Autodesk Inventor part; units mm, degrees
(part 2 of 3)
sketch "Sketch72" plane through (-75.2, 2, 54) normal (0, 1, 0) x (1, 0, 0)
  line L0 (165.4, 13.35) -> (165.4, 23.35) projected
  line L1 (17.3, 78.3) -> (17.3, 97) projected
  line L2 (17.3, 97) -> (-15, 97) projected
  line L3 (-15, 97) -> (-15, 78.3) projected
  line L4 (-15, 78.3) -> (17.3, 78.3) projected
  line L5 (12.24, 7) -> (12.24, 22.5) projected
  line L6 (12.24, 22.5) -> (-7, 22.5) projected
  line L7 (-7, 22.5) -> (-7, 7) projected
  line L8 (-7, 7) -> (12.24, 7) projected
  line L9 (150.4, 110.9) -> (150.4, 105.9) projected
  line L10 (150.4, 105.9) -> (130.4, 105.9) projected
  line L11 (130.4, 105.9) -> (130.4, 110.9) projected
  line L12 (130.4, 110.9) -> (150.4, 110.9) projected
  circle A0 centre (124.902, 56.094) radius 1 projected
  circle A1 centre (89.469, 56.094) radius 1 projected
  circle A2 centre (89.469, 91.502) radius 1 projected
  circle A3 centre (124.902, 91.502) radius 1 projected
  circle A4 centre (104.2, 13.0337) radius 1.5 projected
  circle A5 centre (46.2, 13.0337) radius 1.5 projected
  circle A6 centre (46.2, 36.0337) radius 1.5 projected
  circle A7 centre (104.2, 36.0337) radius 1.5 projected
  circle A8 centre (104.2, 13.0337) radius 3 projected
  circle A9 centre (46.2, 13.0337) radius 3 projected
  circle A10 centre (104.2, 36.0337) radius 3 projected
  circle A11 centre (46.2, 36.0337) radius 3 projected
  circle A12 centre (-2.46, 5.26) radius 1.275 projected
  circle A13 centre (7.7, 5.26) radius 1.275 projected
  line L13 (91.971, 89) -> (91.971, 58.596) projected
  line L14 (91.971, 58.596) -> (102, 58.596) projected
  line L15 (102, 58.596) -> (102, 39.596) projected
  line L16 (102, 39.596) -> (110.4, 39.596) projected
  line L17 (110.4, 39.596) -> (110.4, -1.404) projected
  line L18 (110.4, -1.404) -> (122.4, -1.404) projected
  line L19 (122.4, -1.404) -> (122.4, 56.094) projected
  circle A14 centre (124.902, 56.094) radius 2.502 projected
  line L20 (122.4, 56.094) -> (122.4, 89) projected
  line L21 (122.4, 89) -> (91.971, 89) projected
  circle A15 centre (89.469, 56.094) radius 2.502 projected
  circle A16 centre (124.902, 91.502) radius 2.502 projected
  circle A17 centre (89.469, 91.502) radius 2.502 projected
  line L22 (157.4, 72.95) -> (162.4, 72.95) projected
  line L23 (162.4, 72.95) -> (162.4, 32.95) projected
  line L24 (157.4, 32.95) -> (157.4, 72.95) projected
  line L25 (-7, 72.95) -> (-7, 32.95) projected
  line L26 (-12, 32.95) -> (-12, 72.95) projected
  line L27 (-12, 72.95) -> (-7, 72.95) projected
  line L28 (20, 110.9) -> (20, 105.9) projected
  line L29 (20, 105.9) -> (0, 105.9) projected
  line L30 (0, 105.9) -> (0, 110.9) projected
  line L31 (0, 110.9) -> (20, 110.9) projected
  line L32 (137.4, 37) -> (137.4, 34) projected
  line L33 (137.4, 34) -> (134.2775, 34) projected
  line L34 (134.2775, 34) -> (134.2775, 37) projected
  line L35 (134.2775, 37) -> (137.4, 37) projected
  line L36 (137.4, 37) -> (140.5225, 37) projected
  line L37 (140.5225, 37) -> (140.5225, 34) projected
  line L38 (140.5225, 34) -> (137.4, 34) projected
  arc A18 (-12, 116) -> (-17, 111) centre (-12, 111) ccw projected
  line L39 (-12, 116) -> (36.4, 116) projected
  line L40 (36.4, 116) -> (36.4, 115.5) projected
  line L41 (36.4, 115.5) -> (37, 115.5) projected
  line L42 (37, 115.5) -> (50.2, 115.5) projected
  line L43 (50.2, 115.5) -> (50.8, 115.5) projected
  line L44 (50.8, 115.5) -> (50.8, 116) projected
  line L45 (50.8, 116) -> (60.4, 116) projected
  line L46 (60.4, 116) -> (60.4, 115.5) projected
  line L47 (60.4, 115.5) -> (61, 115.5) projected
  line L48 (61, 115.5) -> (74.2, 115.5) projected
  line L49 (74.2, 115.5) -> (74.8, 115.5) projected
  line L50 (74.8, 115.5) -> (74.8, 116) projected
  line L51 (74.8, 116) -> (162.4, 116) projected
  arc A19 (167.4, 111) -> (162.4, 116) centre (162.4, 111) ccw projected
  line L52 (167.4, 111) -> (167.4, -3) projected
  arc A20 (162.4, -8) -> (167.4, -3) centre (162.4, -3) ccw projected
  line L53 (162.4, -8) -> (-12, -8) projected
  arc A21 (-17, -3) -> (-12, -8) centre (-12, -3) ccw projected
  line L54 (-17, -3) -> (-17, 111) projected
  line L55 (37, 115.5) -> (37, 102.8) projected
  line L56 (37, 102.8) -> (35.5, 102.8) projected
  line L57 (35.5, 102.8) -> (35.5, 112) projected
  line L58 (35.5, 112) -> (34, 112) projected
  line L59 (34, 112) -> (34, 114) projected
  line L60 (34, 114) -> (22, 114) projected
  line L61 (22, 114) -> (22, 112) projected
  line L62 (22, 112) -> (-12, 112) projected
  arc A22 (-12, 112) -> (-13, 111) centre (-12, 111) ccw projected
  line L63 (-13, 111) -> (-13, 100) projected
  line L64 (-13, 100) -> (19.3, 100) projected
  line L65 (19.3, 100) -> (19.3, 75.3) projected
  line L66 (19.3, 75.3) -> (-13, 75.3) projected
  line L67 (-13, 75.3) -> (-13, 77.3) projected
  line L68 (50.2, 102.8) -> (50.2, 115.5) projected
  line L69 (51.7, 102.8) -> (50.2, 102.8) projected
  line L70 (51.7, 112) -> (51.7, 102.8) projected
  line L71 (59.5, 112) -> (51.7, 112) projected
  line L72 (59.5, 102.8) -> (59.5, 112) projected
  line L73 (61, 102.8) -> (59.5, 102.8) projected
  line L74 (61, 115.5) -> (61, 102.8) projected
  line L75 (74.2, 102.8) -> (74.2, 115.5) projected
  line L76 (75.7, 102.8) -> (74.2, 102.8) projected
  line L77 (75.7, 112) -> (75.7, 102.8) projected
  line L78 (116.4, 112) -> (75.7, 112) projected
  line L79 (116.4, 114) -> (116.4, 112) projected
  line L80 (128.4, 114) -> (116.4, 114) projected
  line L81 (128.4, 112) -> (128.4, 114) projected
  line L82 (162.4, 112) -> (128.4, 112) projected
  arc A23 (163.4, 111) -> (162.4, 112) centre (162.4, 111) ccw projected
  line L83 (163.4, -3) -> (163.4, 111) projected
  arc A24 (162.4, -4) -> (163.4, -3) centre (162.4, -3) ccw projected
  line L84 (150.4, -4) -> (162.4, -4) projected
  line L85 (150.4, 0) -> (150.4, -4) projected
  line L86 (130.4, 0) -> (150.4, 0) projected
  line L87 (130.4, -4) -> (130.4, 0) projected
  line L88 (128.4, -4) -> (130.4, -4) projected
  line L89 (128.4, -6) -> (128.4, -4) projected
  line L90 (116.4, -6) -> (128.4, -6) projected
  line L91 (116.4, -4) -> (116.4, -6) projected
  line L92 (34, -4) -> (116.4, -4) projected
  line L93 (34, -4) -> (22, -4) projected
  line L94 (20, -4) -> (22, -4) projected
  line L95 (20, 0) -> (20, -4) projected
  line L96 (0, 0) -> (20, 0) projected
  line L97 (0, -4) -> (0, 0) projected
  line L98 (-12, -4) -> (0, -4) projected
  arc A25 (-13, -3) -> (-12, -4) centre (-12, -3) ccw projected
  line L99 (-13, 48) -> (-13, -3) projected
  line L100 (-13, 48) -> (-13, 60) projected
  line L101 (-13, 75.3) -> (-13, 60) projected
  line L102 (22, 112) -> (34, 112) projected
  line L103 (-13, 98) -> (-13, 100) projected
  line L104 (116.4, 112) -> (128.4, 112) projected
  line L105 (128.4, -4) -> (116.4, -4) projected
  line L106 (34, -6) -> (34, -4) projected
  line L107 (22, -6) -> (34, -6) projected
  line L108 (22, -4) -> (22, -6) projected
  line L109 (-15, 48) -> (-13, 48) projected
  line L110 (-15, 60) -> (-15, 48) projected
  line L111 (-13, 60) -> (-15, 60) projected
  line L112 (163.4, 111) -> (163.4, -3) projected
  line L113 (167.4, 13.35) -> (165.4, 13.35) projected
  line L114 (163.4, 13.35) -> (163.4, 30.0547)
  line L115 (17.3, 78.3) -> (17.3, 97) projected
  line L116 (17.3, 97) -> (-15, 97) projected
  line L117 (-15, 97) -> (-15, 78.3) projected
  line L118 (-15, 78.3) -> (17.3, 78.3) projected
  line L119 (150.4, 110.9) -> (150.4, 105.9) projected
  line L120 (150.4, 105.9) -> (130.4, 105.9) projected
  line L121 (130.4, 105.9) -> (130.4, 110.9) projected
  line L122 (130.4, 110.9) -> (150.4, 110.9) projected
  circle A26 centre (124.902, 56.094) radius 1 projected
  circle A27 centre (89.469, 56.094) radius 1 projected
  circle A28 centre (89.469, 91.502) radius 1 projected
  circle A29 centre (124.902, 91.502) radius 1 projected
  circle A30 centre (104.2, 13.0337) radius 1.5 projected
  circle A31 centre (46.2, 13.0337) radius 1.5 projected
  circle A32 centre (46.2, 36.0337) radius 1.5 projected
  circle A33 centre (104.2, 36.0337) radius 1.5 projected
  circle A34 centre (104.2, 13.0337) radius 3 projected
  circle A35 centre (46.2, 13.0337) radius 3 projected
  circle A36 centre (104.2, 36.0337) radius 3 projected
  circle A37 centre (46.2, 36.0337) radius 3 projected
  circle A38 centre (-2.46, 5.26) radius 1.275 projected
  circle A39 centre (7.7, 5.26) radius 1.275 projected
  line L123 (91.971, 89) -> (91.971, 58.596) projected
  line L124 (91.971, 58.596) -> (102, 58.596) projected
  line L125 (102, 58.596) -> (102, 39.596) projected
  line L126 (102, 39.596) -> (110.4, 39.596) projected
  line L127 (110.4, 39.596) -> (110.4, -1.404) projected
  line L128 (110.4, -1.404) -> (122.4, -1.404) projected
  line L129 (122.4, -1.404) -> (122.4, 56.094) projected
  circle A40 centre (124.902, 56.094) radius 2.502 projected
  line L130 (122.4, 56.094) -> (122.4, 89) projected
  line L131 (122.4, 89) -> (91.971, 89) projected
  circle A41 centre (89.469, 56.094) radius 2.502 projected
  circle A42 centre (124.902, 91.502) radius 2.502 projected
  circle A43 centre (89.469, 91.502) radius 2.502 projected
  line L132 (157.4, 72.95) -> (162.4, 72.95) projected
  line L133 (162.4, 72.95) -> (162.4, 32.95) projected
  line L134 (-12, 32.95) -> (-12, 72.95) projected
  line L135 (-12, 72.95) -> (-7, 72.95) projected
  line L136 (20, 110.9) -> (20, 105.9) projected
  line L137 (20, 105.9) -> (0, 105.9) projected
  line L138 (0, 105.9) -> (0, 110.9) projected
  line L139 (0, 110.9) -> (20, 110.9) projected
  arc A44 (-12, 116) -> (-17, 111) centre (-12, 111) ccw projected
  line L140 (-12, 116) -> (36.4, 116) projected
  line L141 (36.4, 116) -> (36.4, 115.5) projected
  line L142 (36.4, 115.5) -> (37, 115.5) projected
  line L143 (37, 115.5) -> (50.2, 115.5) projected
  line L144 (50.8, 116) -> (60.4, 116) projected
  line L145 (60.4, 116) -> (60.4, 115.5) projected
  line L146 (60.4, 115.5) -> (61, 115.5) projected
  line L147 (61, 115.5) -> (74.2, 115.5) projected
  line L148 (74.8, 116) -> (162.4, 116) projected
  arc A45 (167.4, 111) -> (162.4, 116) centre (162.4, 111) ccw projected
  line L149 (167.4, 111) -> (167.4, -3) projected
  arc A46 (162.4, -8) -> (167.4, -3) centre (162.4, -3) ccw projected
  line L150 (162.4, -8) -> (-12, -8) projected
  arc A47 (-17, -3) -> (-12, -8) centre (-12, -3) ccw projected
  line L151 (-17, -3) -> (-17, 111) projected
  line L152 (37, 115.5) -> (37, 102.8) projected
  line L153 (37, 102.8) -> (35.5, 102.8) projected
  line L154 (35.5, 102.8) -> (35.5, 112) projected
  line L155 (35.5, 112) -> (34, 112) projected
  line L156 (34, 112) -> (34, 114) projected
  line L157 (34, 114) -> (22, 114) projected
  line L158 (22, 114) -> (22, 112) projected
  line L159 (22, 112) -> (-12, 112) projected
  arc A48 (-12, 112) -> (-13, 111) centre (-12, 111) ccw projected
  line L160 (-13, 111) -> (-13, 100) projected
  line L161 (-13, 100) -> (19.3, 100) projected
  line L162 (19.3, 100) -> (19.3, 75.3) projected
  line L163 (19.3, 75.3) -> (-13, 75.3) projected
  line L164 (-13, 75.3) -> (-13, 77.3) projected
  line L165 (59.5, 112) -> (51.7, 112) projected
  line L166 (59.5, 102.8) -> (59.5, 112) projected
  line L167 (61, 102.8) -> (59.5, 102.8) projected
  line L168 (61, 115.5) -> (61, 102.8) projected
  line L169 (116.4, 112) -> (75.7, 112) projected
  line L170 (116.4, 114) -> (116.4, 112) projected
  line L171 (128.4, 114) -> (116.4, 114) projected
  line L172 (128.4, 112) -> (128.4, 114) projected
  line L173 (162.4, 112) -> (128.4, 112) projected
  arc A49 (163.4, 111) -> (162.4, 112) centre (162.4, 111) ccw projected
  line L174 (163.4, -3) -> (163.4, 111) projected
  arc A50 (162.4, -4) -> (163.4, -3) centre (162.4, -3) ccw projected
  line L175 (150.4, -4) -> (162.4, -4) projected
  line L176 (150.4, 0) -> (150.4, -4) projected
  line L177 (130.4, 0) -> (150.4, 0) projected
  line L178 (130.4, -4) -> (130.4, 0) projected
  line L179 (128.4, -4) -> (130.4, -4) projected
  line L180 (128.4, -6) -> (128.4, -4) projected
  line L181 (116.4, -6) -> (128.4, -6) projected
  line L182 (116.4, -4) -> (116.4, -6) projected
  line L183 (34, -4) -> (116.4, -4) projected
  line L184 (34, -4) -> (22, -4) projected
  line L185 (20, -4) -> (22, -4) projected
  line L186 (20, 0) -> (20, -4) projected
  line L187 (0, 0) -> (20, 0) projected
  line L188 (0, -4) -> (0, 0) projected
  line L189 (-12, -4) -> (0, -4) projected
  arc A51 (-13, -3) -> (-12, -4) centre (-12, -3) ccw projected
  line L190 (-13, 48) -> (-13, -3) projected
  line L191 (-13, 48) -> (-13, 60) projected
  line L192 (-13, 75.3) -> (-13, 60) projected
  line L193 (22, 112) -> (34, 112) projected
  line L194 (-13, 98) -> (-13, 100) projected
  line L195 (116.4, 112) -> (128.4, 112) projected
  line L196 (128.4, -4) -> (116.4, -4) projected
  line L197 (34, -6) -> (34, -4) projected
  line L198 (22, -6) -> (34, -6) projected
  line L199 (22, -4) -> (22, -6) projected
  line L200 (-15, 48) -> (-13, 48) projected
  line L201 (-15, 60) -> (-15, 48) projected
  line L202 (-13, 60) -> (-15, 60) projected
  line L203 (17.3, 78.3) -> (17.3, 97) projected
  line L204 (17.3, 97) -> (-15, 97) projected
  line L205 (-15, 97) -> (-15, 78.3) projected
  line L206 (-15, 78.3) -> (17.3, 78.3) projected
  line L207 (150.4, 110.9) -> (150.4, 105.9) projected
  line L208 (150.4, 105.9) -> (130.4, 105.9) projected
  line L209 (130.4, 105.9) -> (130.4, 110.9) projected
  line L210 (130.4, 110.9) -> (150.4, 110.9) projected
  circle A52 centre (124.902, 56.094) radius 1 projected
  circle A53 centre (89.469, 56.094) radius 1 projected
  circle A54 centre (89.469, 91.502) radius 1 projected
  circle A55 centre (124.902, 91.502) radius 1 projected
  circle A56 centre (104.2, 13.0337) radius 1.5 projected
  circle A57 centre (46.2, 13.0337) radius 1.5 projected
  circle A58 centre (46.2, 36.0337) radius 1.5 projected
  circle A59 centre (104.2, 36.0337) radius 1.5 projected
  circle A60 centre (104.2, 13.0337) radius 3 projected
  circle A61 centre (46.2, 13.0337) radius 3 projected
  circle A62 centre (104.2, 36.0337) radius 3 projected
  circle A63 centre (46.2, 36.0337) radius 3 projected
  circle A64 centre (-2.46, 5.26) radius 1.275 projected
  circle A65 centre (7.7, 5.26) radius 1.275 projected
  line L211 (91.971, 89) -> (91.971, 58.596) projected
  line L212 (91.971, 58.596) -> (102, 58.596) projected
  line L213 (102, 58.596) -> (102, 39.596) projected
  line L214 (102, 39.596) -> (110.4, 39.596) projected
  line L215 (110.4, 39.596) -> (110.4, -1.404) projected
  line L216 (110.4, -1.404) -> (122.4, -1.404) projected
  line L217 (122.4, -1.404) -> (122.4, 56.094) projected
  circle A66 centre (124.902, 56.094) radius 2.502 projected
  line L218 (122.4, 56.094) -> (122.4, 89) projected
  line L219 (122.4, 89) -> (91.971, 89) projected
  circle A67 centre (89.469, 56.094) radius 2.502 projected
  circle A68 centre (124.902, 91.502) radius 2.502 projected
  circle A69 centre (89.469, 91.502) radius 2.502 projected
  line L220 (157.4, 72.95) -> (162.4, 72.95) projected
  line L221 (162.4, 72.95) -> (162.4, 32.95) projected
  line L222 (-12, 32.95) -> (-12, 72.95) projected
  line L223 (-12, 72.95) -> (-7, 72.95) projected
  line L224 (20, 110.9) -> (20, 105.9) projected
  line L225 (20, 105.9) -> (0, 105.9) projected
  line L226 (0, 105.9) -> (0, 110.9) projected
  line L227 (0, 110.9) -> (20, 110.9) projected
  arc A70 (-12, 116) -> (-17, 111) centre (-12, 111) ccw projected
  line L228 (-12, 116) -> (36.4, 116) projected
  line L229 (36.4, 116) -> (36.4, 115.5) projected
  line L230 (36.4, 115.5) -> (37, 115.5) projected
  line L231 (37, 115.5) -> (50.2, 115.5) projected
  line L232 (50.8, 116) -> (60.4, 116) projected
  line L233 (60.4, 116) -> (60.4, 115.5) projected
  line L234 (60.4, 115.5) -> (61, 115.5) projected
  line L235 (61, 115.5) -> (74.2, 115.5) projected
  line L236 (74.8, 116) -> (162.4, 116) projected
  arc A71 (167.4, 111) -> (162.4, 116) centre (162.4, 111) ccw projected
  line L237 (167.4, 111) -> (167.4, -3) projected
  arc A72 (162.4, -8) -> (167.4, -3) centre (162.4, -3) ccw projected
  line L238 (162.4, -8) -> (-12, -8) projected
  arc A73 (-17, -3) -> (-12, -8) centre (-12, -3) ccw projected
  line L239 (-17, -3) -> (-17, 111) projected
  line L240 (37, 115.5) -> (37, 102.8) projected
  line L241 (37, 102.8) -> (35.5, 102.8) projected
  line L242 (35.5, 102.8) -> (35.5, 112) projected
  line L243 (35.5, 112) -> (34, 112) projected
  line L244 (34, 112) -> (34, 114) projected
  line L245 (34, 114) -> (22, 114) projected
  line L246 (22, 114) -> (22, 112) projected
  line L247 (22, 112) -> (-12, 112) projected
  arc A74 (-12, 112) -> (-13, 111) centre (-12, 111) ccw projected
  line L248 (-13, 111) -> (-13, 100) projected
  line L249 (-13, 100) -> (19.3, 100) projected
  line L250 (19.3, 100) -> (19.3, 75.3) projected
  line L251 (19.3, 75.3) -> (-13, 75.3) projected
  line L252 (-13, 75.3) -> (-13, 77.3) projected
  line L253 (59.5, 112) -> (51.7, 112) projected
  line L254 (59.5, 102.8) -> (59.5, 112) projected
  line L255 (61, 102.8) -> (59.5, 102.8) projected
  line L256 (61, 115.5) -> (61, 102.8) projected
  line L257 (116.4, 112) -> (75.7, 112) projected
  line L258 (116.4, 114) -> (116.4, 112) projected
  line L259 (128.4, 114) -> (116.4, 114) projected
  line L260 (128.4, 112) -> (128.4, 114) projected
  line L261 (162.4, 112) -> (128.4, 112) projected
  arc A75 (163.4, 111) -> (162.4, 112) centre (162.4, 111) ccw projected
  line L262 (163.4, -3) -> (163.4, 111) projected
  arc A76 (162.4, -4) -> (163.4, -3) centre (162.4, -3) ccw projected
  line L263 (150.4, -4) -> (162.4, -4) projected
  line L264 (150.4, 0) -> (150.4, -4) projected
  line L265 (130.4, 0) -> (150.4, 0) projected
  line L266 (130.4, -4) -> (130.4, 0) projected
  line L267 (128.4, -4) -> (130.4, -4) projected
  line L268 (128.4, -6) -> (128.4, -4) projected
  line L269 (116.4, -6) -> (128.4, -6) projected
  line L270 (116.4, -4) -> (116.4, -6) projected
  line L271 (34, -4) -> (116.4, -4) projected
  line L272 (34, -4) -> (22, -4) projected
  line L273 (20, -4) -> (22, -4) projected
  line L274 (20, 0) -> (20, -4) projected
  line L275 (0, 0) -> (20, 0) projected
  line L276 (0, -4) -> (0, 0) projected
  line L277 (-12, -4) -> (0, -4) projected
  arc A77 (-13, -3) -> (-12, -4) centre (-12, -3) ccw projected
  line L278 (-13, 48) -> (-13, -3) projected
  line L279 (-13, 48) -> (-13, 60) projected
  line L280 (-13, 75.3) -> (-13, 60) projected
  line L281 (22, 112) -> (34, 112) projected
  line L282 (-13, 98) -> (-13, 100) projected
  line L283 (116.4, 112) -> (128.4, 112) projected
  line L284 (128.4, -4) -> (116.4, -4) projected
  line L285 (34, -6) -> (34, -4) projected
  line L286 (22, -6) -> (34, -6) projected
  line L287 (22, -4) -> (22, -6) projected
  line L288 (-15, 48) -> (-13, 48) projected
  line L289 (-15, 60) -> (-15, 48) projected
  line L290 (-13, 60) -> (-15, 60) projected
  line L291 (17.3, 78.3) -> (17.3, 97) projected
  line L292 (17.3, 97) -> (-15, 97) projected
  line L293 (-15, 97) -> (-15, 78.3) projected
  line L294 (-15, 78.3) -> (17.3, 78.3) projected
  line L295 (150.4, 110.9) -> (150.4, 105.9) projected
  line L296 (150.4, 105.9) -> (130.4, 105.9) projected
  line L297 (130.4, 105.9) -> (130.4, 110.9) projected
  line L298 (130.4, 110.9) -> (150.4, 110.9) projected
  circle A78 centre (124.902, 56.094) radius 1 projected
  circle A79 centre (89.469, 56.094) radius 1 projected
  circle A80 centre (89.469, 91.502) radius 1 projected
  circle A81 centre (124.902, 91.502) radius 1 projected
  circle A82 centre (104.2, 13.0337) radius 1.5 projected
  circle A83 centre (46.2, 13.0337) radius 1.5 projected
  circle A84 centre (46.2, 36.0337) radius 1.5 projected
  circle A85 centre (104.2, 36.0337) radius 1.5 projected
  circle A86 centre (104.2, 13.0337) radius 3 projected
  circle A87 centre (46.2, 13.0337) radius 3 projected
  circle A88 centre (104.2, 36.0337) radius 3 projected
  circle A89 centre (46.2, 36.0337) radius 3 projected
  circle A90 centre (-2.46, 5.26) radius 1.275 projected
  circle A91 centre (7.7, 5.26) radius 1.275 projected
  line L299 (91.971, 89) -> (91.971, 58.596) projected
  line L300 (91.971, 58.596) -> (102, 58.596) projected
  line L301 (102, 58.596) -> (102, 39.596) projected
  line L302 (102, 39.596) -> (110.4, 39.596) projected
  line L303 (110.4, 39.596) -> (110.4, -1.404) projected
  line L304 (110.4, -1.404) -> (122.4, -1.404) projected
  line L305 (122.4, -1.404) -> (122.4, 56.094) projected
  circle A92 centre (124.902, 56.094) radius 2.502 projected
  line L306 (122.4, 56.094) -> (122.4, 89) projected
  line L307 (122.4, 89) -> (91.971, 89) projected
  circle A93 centre (89.469, 56.094) radius 2.502 projected
  circle A94 centre (124.902, 91.502) radius 2.502 projected
  circle A95 centre (89.469, 91.502) radius 2.502 projected
  line L308 (157.4, 72.95) -> (162.4, 72.95) projected
  line L309 (162.4, 72.95) -> (162.4, 32.95) projected
  line L310 (-12, 32.95) -> (-12, 72.95) projected
  line L311 (-12, 72.95) -> (-7, 72.95) projected
  line L312 (20, 110.9) -> (20, 105.9) projected
  line L313 (20, 105.9) -> (0, 105.9) projected
  line L314 (0, 105.9) -> (0, 110.9) projected
  line L315 (0, 110.9) -> (20, 110.9) projected
  arc A96 (-12, 116) -> (-17, 111) centre (-12, 111) ccw projected
  line L316 (-12, 116) -> (36.4, 116) projected
  line L317 (36.4, 116) -> (36.4, 115.5) projected
  line L318 (36.4, 115.5) -> (37, 115.5) projected
  line L319 (37, 115.5) -> (50.2, 115.5) projected
  line L320 (50.8, 116) -> (60.4, 116) projected
  line L321 (60.4, 116) -> (60.4, 115.5) projected
  line L322 (60.4, 115.5) -> (61, 115.5) projected
  line L323 (61, 115.5) -> (74.2, 115.5) projected
  line L324 (74.8, 116) -> (162.4, 116) projected
  arc A97 (167.4, 111) -> (162.4, 116) centre (162.4, 111) ccw projected
  line L325 (167.4, 111) -> (167.4, -3) projected
  arc A98 (162.4, -8) -> (167.4, -3) centre (162.4, -3) ccw projected
  line L326 (162.4, -8) -> (-12, -8) projected
  arc A99 (-17, -3) -> (-12, -8) centre (-12, -3) ccw projected
  line L327 (-17, -3) -> (-17, 111) projected
  line L328 (37, 115.5) -> (37, 102.8) projected
  line L329 (37, 102.8) -> (35.5, 102.8) projected
  line L330 (35.5, 102.8) -> (35.5, 112) projected
  line L331 (35.5, 112) -> (34, 112) projected
  line L332 (34, 112) -> (34, 114) projected
  line L333 (34, 114) -> (22, 114) projected
  line L334 (22, 114) -> (22, 112) projected
  line L335 (22, 112) -> (-12, 112) projected
  arc A100 (-12, 112) -> (-13, 111) centre (-12, 111) ccw projected
  line L336 (-13, 111) -> (-13, 100) projected
  line L337 (-13, 100) -> (19.3, 100) projected
  line L338 (19.3, 100) -> (19.3, 75.3) projected
  line L339 (19.3, 75.3) -> (-13, 75.3) projected
  line L340 (-13, 75.3) -> (-13, 77.3) projected
  line L341 (59.5, 112) -> (51.7, 112) projected
  line L342 (59.5, 102.8) -> (59.5, 112) projected
  line L343 (61, 102.8) -> (59.5, 102.8) projected
  line L344 (61, 115.5) -> (61, 102.8) projected
  line L345 (116.4, 112) -> (75.7, 112) projected
  line L346 (116.4, 114) -> (116.4, 112) projected
  line L347 (128.4, 114) -> (116.4, 114) projected
  line L348 (128.4, 112) -> (128.4, 114) projected
  line L349 (162.4, 112) -> (128.4, 112) projected
  arc A101 (163.4, 111) -> (162.4, 112) centre (162.4, 111) ccw projected
  line L350 (163.4, -3) -> (163.4, 111) projected
  arc A102 (162.4, -4) -> (163.4, -3) centre (162.4, -3) ccw projected
  line L351 (150.4, -4) -> (162.4, -4) projected
  line L352 (150.4, 0) -> (150.4, -4) projected
  line L353 (130.4, 0) -> (150.4, 0) projected
  line L354 (130.4, -4) -> (130.4, 0) projected
  line L355 (128.4, -4) -> (130.4, -4) projected
  line L356 (128.4, -6) -> (128.4, -4) projected
  line L357 (116.4, -6) -> (128.4, -6) projected
  line L358 (116.4, -4) -> (116.4, -6) projected
  line L359 (34, -4) -> (116.4, -4) projected
  line L360 (34, -4) -> (22, -4) projected
  line L361 (20, -4) -> (22, -4) projected
  line L362 (20, 0) -> (20, -4) projected
  line L363 (0, 0) -> (20, 0) projected
  line L364 (0, -4) -> (0, 0) projected
  line L365 (-12, -4) -> (0, -4) projected
  arc A103 (-13, -3) -> (-12, -4) centre (-12, -3) ccw projected
  line L366 (-13, 48) -> (-13, -3) projected
  line L367 (-13, 48) -> (-13, 60) projected
  line L368 (-13, 75.3) -> (-13, 60) projected
  line L369 (22, 112) -> (34, 112) projected
  line L370 (-13, 98) -> (-13, 100) projected
  line L371 (116.4, 112) -> (128.4, 112) projected
  line L372 (128.4, -4) -> (116.4, -4) projected
  line L373 (34, -6) -> (34, -4) projected
  line L374 (22, -6) -> (34, -6) projected
  line L375 (22, -4) -> (22, -6) projected
  line L376 (-15, 48) -> (-13, 48) projected
  line L377 (-15, 60) -> (-15, 48) projected
  line L378 (-13, 60) -> (-15, 60) projected
  line L379 (17.3, 78.3) -> (17.3, 97) projected
  line L380 (17.3, 97) -> (-15, 97) projected
  line L381 (-15, 97) -> (-15, 78.3) projected
  line L382 (-15, 78.3) -> (17.3, 78.3) projected
  line L383 (150.4, 110.9) -> (150.4, 105.9) projected
  line L384 (150.4, 105.9) -> (130.4, 105.9) projected
  line L385 (130.4, 105.9) -> (130.4, 110.9) projected
  line L386 (130.4, 110.9) -> (150.4, 110.9) projected
  circle A104 centre (124.902, 56.094) radius 1 projected
  circle A105 centre (89.469, 56.094) radius 1 projected
  circle A106 centre (89.469, 91.502) radius 1 projected
  circle A107 centre (124.902, 91.502) radius 1 projected
  circle A108 centre (104.2, 13.0337) radius 1.5 projected
  circle A109 centre (46.2, 13.0337) radius 1.5 projected
  circle A110 centre (46.2, 36.0337) radius 1.5 projected
  circle A111 centre (104.2, 36.0337) radius 1.5 projected
  circle A112 centre (104.2, 13.0337) radius 3 projected
  circle A113 centre (46.2, 13.0337) radius 3 projected
  circle A114 centre (104.2, 36.0337) radius 3 projected
  circle A115 centre (46.2, 36.0337) radius 3 projected
  circle A116 centre (-2.46, 5.26) radius 1.275 projected
  circle A117 centre (7.7, 5.26) radius 1.275 projected
  line L387 (91.971, 89) -> (91.971, 58.596) projected
  line L388 (91.971, 58.596) -> (102, 58.596) projected
  line L389 (102, 58.596) -> (102, 39.596) projected
  line L390 (102, 39.596) -> (110.4, 39.596) projected
  line L391 (110.4, 39.596) -> (110.4, -1.404) projected
  line L392 (110.4, -1.404) -> (122.4, -1.404) projected
  line L393 (122.4, -1.404) -> (122.4, 56.094) projected
  circle A118 centre (124.902, 56.094) radius 2.502 projected
  line L394 (122.4, 56.094) -> (122.4, 89) projected
  line L395 (122.4, 89) -> (91.971, 89) projected
  circle A119 centre (89.469, 56.094) radius 2.502 projected
  circle A120 centre (124.902, 91.502) radius 2.502 projected
  circle A121 centre (89.469, 91.502) radius 2.502 projected
  line L396 (157.4, 72.95) -> (162.4, 72.95) projected
  line L397 (162.4, 72.95) -> (162.4, 32.95) projected
  line L398 (-12, 32.95) -> (-12, 72.95) projected
  line L399 (-12, 72.95) -> (-7, 72.95) projected
  line L400 (20, 110.9) -> (20, 105.9) projected
  line L401 (20, 105.9) -> (0, 105.9) projected
  line L402 (0, 105.9) -> (0, 110.9) projected
  line L403 (0, 110.9) -> (20, 110.9) projected
  arc A122 (-12, 116) -> (-17, 111) centre (-12, 111) ccw projected
  line L404 (-12, 116) -> (36.4, 116) projected
  line L405 (36.4, 116) -> (36.4, 115.5) projected
  line L406 (36.4, 115.5) -> (37, 115.5) projected
  line L407 (37, 115.5) -> (50.2, 115.5) projected
  line L408 (50.8, 116) -> (60.4, 116) projected
  line L409 (60.4, 116) -> (60.4, 115.5) projected
  line L410 (60.4, 115.5) -> (61, 115.5) projected
  line L411 (61, 115.5) -> (74.2, 115.5) projected
  line L412 (74.8, 116) -> (162.4, 116) projected
  arc A123 (167.4, 111) -> (162.4, 116) centre (162.4, 111) ccw projected
  line L413 (167.4, 111) -> (167.4, -3) projected
  arc A124 (162.4, -8) -> (167.4, -3) centre (162.4, -3) ccw projected
  line L414 (162.4, -8) -> (-12, -8) projected
  arc A125 (-17, -3) -> (-12, -8) centre (-12, -3) ccw projected
  line L415 (-17, -3) -> (-17, 111) projected
  line L416 (37, 115.5) -> (37, 102.8) projected
  line L417 (37, 102.8) -> (35.5, 102.8) projected
  line L418 (35.5, 102.8) -> (35.5, 112) projected
  line L419 (35.5, 112) -> (34, 112) projected
  line L420 (34, 112) -> (34, 114) projected
  line L421 (34, 114) -> (22, 114) projected
  line L422 (22, 114) -> (22, 112) projected
  line L423 (22, 112) -> (-12, 112) projected
  arc A126 (-12, 112) -> (-13, 111) centre (-12, 111) ccw projected
  line L424 (-13, 111) -> (-13, 100) projected
  line L425 (-13, 100) -> (19.3, 100) projected
  line L426 (19.3, 100) -> (19.3, 75.3) projected
  line L427 (19.3, 75.3) -> (-13, 75.3) projected
  line L428 (-13, 75.3) -> (-13, 77.3) projected
  line L429 (59.5, 112) -> (51.7, 112) projected
  line L430 (59.5, 102.8) -> (59.5, 112) projected
  line L431 (61, 102.8) -> (59.5, 102.8) projected
  line L432 (61, 115.5) -> (61, 102.8) projected
  line L433 (116.4, 112) -> (75.7, 112) projected
  line L434 (116.4, 114) -> (116.4, 112) projected
  line L435 (128.4, 114) -> (116.4, 114) projected
  line L436 (128.4, 112) -> (128.4, 114) projected
  line L437 (162.4, 112) -> (128.4, 112) projected
  arc A127 (163.4, 111) -> (162.4, 112) centre (162.4, 111) ccw projected
  line L438 (163.4, -3) -> (163.4, 111) projected
  arc A128 (162.4, -4) -> (163.4, -3) centre (162.4, -3) ccw projected
  line L439 (150.4, -4) -> (162.4, -4) projected
  line L440 (150.4, 0) -> (150.4, -4) projected
  line L441 (130.4, 0) -> (150.4, 0) projected
  line L442 (130.4, -4) -> (130.4, 0) projected
  line L443 (128.4, -4) -> (130.4, -4) projected
  line L444 (128.4, -6) -> (128.4, -4) projected
  line L445 (116.4, -6) -> (128.4, -6) projected
  line L446 (116.4, -4) -> (116.4, -6) projected
  line L447 (34, -4) -> (116.4, -4) projected
  line L448 (34, -4) -> (22, -4) projected
  line L449 (20, -4) -> (22, -4) projected
  line L450 (20, 0) -> (20, -4) projected
  line L451 (0, 0) -> (20, 0) projected
  line L452 (0, -4) -> (0, 0) projected
  line L453 (-12, -4) -> (0, -4) projected
  arc A129 (-13, -3) -> (-12, -4) centre (-12, -3) ccw projected
  line L454 (-13, 48) -> (-13, -3) projected
  line L455 (-13, 48) -> (-13, 60) projected
  line L456 (-13, 75.3) -> (-13, 60) projected
  line L457 (22, 112) -> (34, 112) projected
  line L458 (-13, 98) -> (-13, 100) projected
  line L459 (116.4, 112) -> (128.4, 112) projected
  line L460 (128.4, -4) -> (116.4, -4) projected
  line L461 (34, -6) -> (34, -4) projected
  line L462 (22, -6) -> (34, -6) projected
  line L463 (22, -4) -> (22, -6) projected
  line L464 (-15, 48) -> (-13, 48) projected
  line L465 (-15, 60) -> (-15, 48) projected
  line L466 (-13, 60) -> (-15, 60) projected
  line L467 (17.3, 78.3) -> (17.3, 97) projected
  line L468 (17.3, 97) -> (-15, 97) projected
  line L469 (-15, 97) -> (-15, 78.3) projected
  line L470 (-15, 78.3) -> (17.3, 78.3) projected
  line L471 (150.4, 110.9) -> (150.4, 105.9) projected
  line L472 (150.4, 105.9) -> (130.4, 105.9) projected
  line L473 (130.4, 105.9) -> (130.4, 110.9) projected
  line L474 (130.4, 110.9) -> (150.4, 110.9) projected
  circle A130 centre (124.902, 56.094) radius 1 projected
  circle A131 centre (89.469, 56.094) radius 1 projected
  circle A132 centre (89.469, 91.502) radius 1 projected
  circle A133 centre (124.902, 91.502) radius 1 projected
  circle A134 centre (104.2, 13.0337) radius 1.5 projected
  circle A135 centre (46.2, 13.0337) radius 1.5 projected
  circle A136 centre (46.2, 36.0337) radius 1.5 projected
  circle A137 centre (104.2, 36.0337) radius 1.5 projected
  circle A138 centre (104.2, 13.0337) radius 3 projected
  circle A139 centre (46.2, 13.0337) radius 3 projected
  circle A140 centre (104.2, 36.0337) radius 3 projected
  circle A141 centre (46.2, 36.0337) radius 3 projected
  circle A142 centre (-2.46, 5.26) radius 1.275 projected
  circle A143 centre (7.7, 5.26) radius 1.275 projected
  line L475 (91.971, 89) -> (91.971, 58.596) projected
  line L476 (91.971, 58.596) -> (102, 58.596) projected
  line L477 (102, 58.596) -> (102, 39.596) projected
  line L478 (102, 39.596) -> (110.4, 39.596) projected
  line L479 (110.4, 39.596) -> (110.4, -1.404) projected
  line L480 (110.4, -1.404) -> (122.4, -1.404) projected
  line L481 (122.4, -1.404) -> (122.4, 56.094) projected
  circle A144 centre (124.902, 56.094) radius 2.502 projected
  line L482 (122.4, 56.094) -> (122.4, 89) projected
  line L483 (122.4, 89) -> (91.971, 89) projected
  circle A145 centre (89.469, 56.094) radius 2.502 projected
  circle A146 centre (124.902, 91.502) radius 2.502 projected
  circle A147 centre (89.469, 91.502) radius 2.502 projected
  line L484 (157.4, 72.95) -> (162.4, 72.95) projected
  line L485 (162.4, 72.95) -> (162.4, 32.95) projected
  line L486 (-12, 32.95) -> (-12, 72.95) projected
  line L487 (-12, 72.95) -> (-7, 72.95) projected
  line L488 (20, 110.9) -> (20, 105.9) projected
  line L489 (20, 105.9) -> (0, 105.9) projected
  line L490 (0, 105.9) -> (0, 110.9) projected
  line L491 (0, 110.9) -> (20, 110.9) projected
  arc A148 (-12, 116) -> (-17, 111) centre (-12, 111) ccw projected
  line L492 (-12, 116) -> (36.4, 116) projected
  line L493 (36.4, 116) -> (36.4, 115.5) projected
  line L494 (36.4, 115.5) -> (37, 115.5) projected
  line L495 (37, 115.5) -> (50.2, 115.5) projected
  line L496 (50.8, 116) -> (60.4, 116) projected
  line L497 (60.4, 116) -> (60.4, 115.5) projected
  line L498 (60.4, 115.5) -> (61, 115.5) projected
  line L499 (61, 115.5) -> (74.2, 115.5) projected
  line L500 (74.8, 116) -> (162.4, 116) projected
  arc A149 (167.4, 111) -> (162.4, 116) centre (162.4, 111) ccw projected
  line L501 (167.4, 111) -> (167.4, -3) projected
  arc A150 (162.4, -8) -> (167.4, -3) centre (162.4, -3) ccw projected
  line L502 (162.4, -8) -> (-12, -8) projected
  arc A151 (-17, -3) -> (-12, -8) centre (-12, -3) ccw projected
  line L503 (-17, -3) -> (-17, 111) projected
  line L504 (37, 115.5) -> (37, 102.8) projected
  line L505 (37, 102.8) -> (35.5, 102.8) projected
  line L506 (35.5, 102.8) -> (35.5, 112) projected
  line L507 (35.5, 112) -> (34, 112) projected
  line L508 (34, 112) -> (34, 114) projected
  line L509 (34, 114) -> (22, 114) projected
  line L510 (22, 114) -> (22, 112) projected
  line L511 (22, 112) -> (-12, 112) projected
  arc A152 (-12, 112) -> (-13, 111) centre (-12, 111) ccw projected
  line L512 (-13, 111) -> (-13, 100) projected
  line L513 (-13, 100) -> (19.3, 100) projected
  line L514 (19.3, 100) -> (19.3, 75.3) projected
  line L515 (19.3, 75.3) -> (-13, 75.3) projected
  line L516 (-13, 75.3) -> (-13, 77.3) projected
  line L517 (59.5, 112) -> (51.7, 112) projected
  line L518 (59.5, 102.8) -> (59.5, 112) projected
  line L519 (61, 102.8) -> (59.5, 102.8) projected
  line L520 (61, 115.5) -> (61, 102.8) projected
  line L521 (116.4, 112) -> (75.7, 112) projected
  line L522 (116.4, 114) -> (116.4, 112) projected
  line L523 (128.4, 114) -> (116.4, 114) projected
  line L524 (128.4, 112) -> (128.4, 114) projected
  line L525 (162.4, 112) -> (128.4, 112) projected
  arc A153 (163.4, 111) -> (162.4, 112) centre (162.4, 111) ccw projected
  line L526 (163.4, -3) -> (163.4, 111) projected
  arc A154 (162.4, -4) -> (163.4, -3) centre (162.4, -3) ccw projected
  line L527 (150.4, -4) -> (162.4, -4) projected
  line L528 (150.4, 0) -> (150.4, -4) projected
  line L529 (130.4, 0) -> (150.4, 0) projected
  line L530 (130.4, -4) -> (130.4, 0) projected
  line L531 (128.4, -4) -> (130.4, -4) projected
  line L532 (128.4, -6) -> (128.4, -4) projected
  line L533 (116.4, -6) -> (128.4, -6) projected
  line L534 (116.4, -4) -> (116.4, -6) projected
  line L535 (34, -4) -> (116.4, -4) projected
  line L536 (34, -4) -> (22, -4) projected
  line L537 (20, -4) -> (22, -4) projected
  line L538 (20, 0) -> (20, -4) projected
  line L539 (0, 0) -> (20, 0) projected
  line L540 (0, -4) -> (0, 0) projected
  line L541 (-12, -4) -> (0, -4) projected
  arc A155 (-13, -3) -> (-12, -4) centre (-12, -3) ccw projected
  line L542 (-13, 48) -> (-13, -3) projected
  line L543 (-13, 48) -> (-13, 60) projected
  line L544 (-13, 75.3) -> (-13, 60) projected
  line L545 (22, 112) -> (34, 112) projected
  line L546 (-13, 98) -> (-13, 100) projected
  line L547 (116.4, 112) -> (128.4, 112) projected
  line L548 (128.4, -4) -> (116.4, -4) projected
  line L549 (34, -6) -> (34, -4) projected
  line L550 (22, -6) -> (34, -6) projected
  line L551 (22, -4) -> (22, -6) projected
  line L552 (-15, 48) -> (-13, 48) projected
  line L553 (-15, 60) -> (-15, 48) projected
  line L554 (-13, 60) -> (-15, 60) projected
  line L555 (167.4, 28.7) -> (165.4, 28.7) projected
  line L556 (167.4, 13.35) -> (165.4, 13.35) projected
  line L557 (165.4, 32.8951) -> (163.4, 32.8951)
  line L558 (163.4, 32.8951) -> (163.4, -2.2797)
  line L559 (163.4, -2.2797) -> (165.4, -2.2797)
  line L560 (165.4, -2.2797) -> (165.4, 32.8951)
  line L561 (12.24, 7) -> (12.24, 22.5) projected
  line L562 (12.24, 22.5) -> (-7, 22.5) projected
  line L563 (-7, 22.5) -> (-7, 7) projected
  line L564 (-7, 7) -> (12.24, 7) projected
  line L565 (50.2, 115.5) -> (50.8, 115.5) projected
  line L566 (50.8, 115.5) -> (50.8, 116) projected
  line L567 (74.2, 115.5) -> (74.8, 115.5) projected
  line L568 (74.8, 115.5) -> (74.8, 116) projected
  line L569 (50.2, 102.8) -> (50.2, 115.5) projected
  line L570 (51.7, 102.8) -> (50.2, 102.8) projected
  line L571 (51.7, 112) -> (51.7, 102.8) projected
  line L572 (74.2, 102.8) -> (74.2, 115.5) projected
  line L573 (75.7, 102.8) -> (74.2, 102.8) projected
  line L574 (75.7, 112) -> (75.7, 102.8) projected
  line L575 (50.2, 115.5) -> (50.8, 115.5) projected
  line L576 (50.8, 115.5) -> (50.8, 116) projected
  line L577 (74.2, 115.5) -> (74.8, 115.5) projected
  line L578 (74.8, 115.5) -> (74.8, 116) projected
  line L579 (50.2, 102.8) -> (50.2, 115.5) projected
  line L580 (51.7, 102.8) -> (50.2, 102.8) projected
  line L581 (51.7, 112) -> (51.7, 102.8) projected
  line L582 (74.2, 102.8) -> (74.2, 115.5) projected
  line L583 (75.7, 102.8) -> (74.2, 102.8) projected
  line L584 (75.7, 112) -> (75.7, 102.8) projected
  line L585 (50.2, 115.5) -> (50.8, 115.5) projected
  line L586 (50.8, 115.5) -> (50.8, 116) projected
  line L587 (74.2, 115.5) -> (74.8, 115.5) projected
  line L588 (74.8, 115.5) -> (74.8, 116) projected
  line L589 (50.2, 102.8) -> (50.2, 115.5) projected
  line L590 (51.7, 102.8) -> (50.2, 102.8) projected
  line L591 (51.7, 112) -> (51.7, 102.8) projected
  line L592 (74.2, 102.8) -> (74.2, 115.5) projected
  line L593 (75.7, 102.8) -> (74.2, 102.8) projected
  line L594 (75.7, 112) -> (75.7, 102.8) projected
  line L595 (50.2, 115.5) -> (50.8, 115.5) projected
  line L596 (50.8, 115.5) -> (50.8, 116) projected
  line L597 (74.2, 115.5) -> (74.8, 115.5) projected
  line L598 (74.8, 115.5) -> (74.8, 116) projected
  line L599 (50.2, 102.8) -> (50.2, 115.5) projected
  line L600 (51.7, 102.8) -> (50.2, 102.8) projected
  line L601 (51.7, 112) -> (51.7, 102.8) projected
  line L602 (74.2, 102.8) -> (74.2, 115.5) projected
  line L603 (75.7, 102.8) -> (74.2, 102.8) projected
  line L604 (75.7, 112) -> (75.7, 102.8) projected
  line L605 (50.2, 115.5) -> (50.8, 115.5) projected
  line L606 (50.8, 115.5) -> (50.8, 116) projected
  line L607 (74.2, 115.5) -> (74.8, 115.5) projected
  line L608 (74.8, 115.5) -> (74.8, 116) projected
  line L609 (50.2, 102.8) -> (50.2, 115.5) projected
  line L610 (51.7, 102.8) -> (50.2, 102.8) projected
  line L611 (51.7, 112) -> (51.7, 102.8) projected
  line L612 (74.2, 102.8) -> (74.2, 115.5) projected
  line L613 (75.7, 102.8) -> (74.2, 102.8) projected
  line L614 (75.7, 112) -> (75.7, 102.8) projected
  line L615 (162.4, 32.95) -> (157.4, 32.95) projected
  line L616 (157.4, 32.95) -> (157.4, 72.95) projected
  line L617 (-7, 72.95) -> (-7, 32.95) projected
  line L618 (-7, 32.95) -> (-12, 32.95) projected
  line L619 (162.4, 32.95) -> (157.4, 32.95) projected
  line L620 (157.4, 32.95) -> (157.4, 72.95) projected
  line L621 (-7, 72.95) -> (-7, 32.95) projected
  line L622 (-7, 32.95) -> (-12, 32.95) projected
  line L623 (162.4, 32.95) -> (157.4, 32.95) projected
  line L624 (157.4, 32.95) -> (157.4, 72.95) projected
  line L625 (-7, 72.95) -> (-7, 32.95) projected
  line L626 (-7, 32.95) -> (-12, 32.95) projected
  line L627 (162.4, 32.95) -> (157.4, 32.95) projected
  line L628 (157.4, 32.95) -> (157.4, 72.95) projected
  line L629 (-7, 72.95) -> (-7, 32.95) projected
  line L630 (-7, 32.95) -> (-12, 32.95) projected
  line L631 (162.4, 32.95) -> (157.4, 32.95) projected
  line L632 (157.4, 32.95) -> (157.4, 72.95) projected
  line L633 (-7, 72.95) -> (-7, 32.95) projected
  line L634 (-7, 32.95) -> (-12, 32.95) projected
  line L635 (162.4, 32.95) -> (157.4, 32.95) projected
  line L636 (-7, 32.95) -> (-12, 32.95) projected
  line L637 (137.4, 37) -> (137.4, 34) projected
  line L638 (137.4, 34) -> (134.2775, 34) projected
  line L639 (134.2775, 34) -> (134.2775, 37) projected
  line L640 (134.2775, 37) -> (137.4, 37) projected
  line L641 (137.4, 37) -> (140.5225, 37) projected
  line L642 (140.5225, 37) -> (140.5225, 34) projected
  line L643 (140.5225, 34) -> (137.4, 34) projected
  line L644 (12.24, 7) -> (12.24, 22.5) projected
  line L645 (12.24, 22.5) -> (-7, 22.5) projected
  line L646 (-7, 22.5) -> (-7, 7) projected
  line L647 (-7, 7) -> (12.24, 7) projected
  line L648 (137.4, 37) -> (137.4, 34) projected
  line L649 (137.4, 34) -> (134.2775, 34) projected
  line L650 (134.2775, 34) -> (134.2775, 37) projected
  line L651 (134.2775, 37) -> (137.4, 37) projected
  line L652 (137.4, 37) -> (140.5225, 37) projected
  line L653 (140.5225, 37) -> (140.5225, 34) projected
  line L654 (140.5225, 34) -> (137.4, 34) projected
  line L655 (12.24, 7) -> (12.24, 22.5) projected
  line L656 (12.24, 22.5) -> (-7, 22.5) projected
  line L657 (-7, 22.5) -> (-7, 7) projected
  line L658 (-7, 7) -> (12.24, 7) projected
  line L659 (137.4, 37) -> (137.4, 34) projected
  line L660 (137.4, 34) -> (134.2775, 34) projected
  line L661 (134.2775, 34) -> (134.2775, 37) projected
  line L662 (134.2775, 37) -> (137.4, 37) projected
  line L663 (137.4, 37) -> (140.5225, 37) projected
  line L664 (140.5225, 37) -> (140.5225, 34) projected
  line L665 (140.5225, 34) -> (137.4, 34) projected
  line L666 (12.24, 7) -> (12.24, 22.5) projected
  line L667 (12.24, 22.5) -> (-7, 22.5) projected
  line L668 (-7, 22.5) -> (-7, 7) projected
  line L669 (-7, 7) -> (12.24, 7) projected
  line L670 (137.4, 37) -> (137.4, 34) projected
  line L671 (137.4, 34) -> (134.2775, 34) projected
  line L672 (134.2775, 34) -> (134.2775, 37) projected
  line L673 (134.2775, 37) -> (137.4, 37) projected
  line L674 (137.4, 37) -> (140.5225, 37) projected
  line L675 (140.5225, 37) -> (140.5225, 34) projected
  line L676 (140.5225, 34) -> (137.4, 34) projected
  line L677 (12.24, 7) -> (12.24, 22.5) projected
  line L678 (12.24, 22.5) -> (-7, 22.5) projected
  line L679 (-7, 22.5) -> (-7, 7) projected
  line L680 (-7, 7) -> (12.24, 7) projected
  line L681 (137.4, 37) -> (137.4, 34) projected
  line L682 (137.4, 34) -> (134.2775, 34) projected
  line L683 (134.2775, 34) -> (134.2775, 37) projected
  line L684 (134.2775, 37) -> (137.4, 37) projected
  line L685 (137.4, 37) -> (140.5225, 37) projected
  line L686 (140.5225, 37) -> (140.5225, 34) projected
  line L687 (140.5225, 34) -> (137.4, 34) projected
  point P0 (75.2, 54)
  point P1 (163.4, -2.2797)
  point P2 (6.9482, 0)
  dimension "d461" = 2
  dimension "d462" = 35.1748
  constraints: 10 end point, 6 horizontal alignment, 2 parallel, 2 point on line, 1 horizontal, 1 perpendicular
  measures "d461" distance of L558.end L559.end
  measures "d462" distance of L559.end L557.start
extrude "Extrusion60" cut sketch "Sketch72" along normal blind 2 contours L560 L559 L83 L557 L0
mirror "Mirror24" about plane through (0, 0, 0) normal (1, 0, 0) of "Extrusion40"
chamfer "Chamfer12" distance 1 angle 45 1 edges at (-72.05, 2, -21.3)
chamfer "Chamfer13" distance 1 angle 45 3 edges at (-55.9, 2, -20.8) (-55.9, 2, -33.65) (-72.05, 2, -46)
chamfer "Chamfer14" distance 1 angle 45 2 edges at (-31.6, 9.2, -60) (-7.6, 9.2, -60)
mirror "Mirror25" about plane through (0, 0, 0) normal (1, 0, 0) of "Extrusion33"
sketch "Sketch75" plane through (-75.2, 2, 54) normal (0, 1, 0) x (1, 0, 0)
  line L0 (17.3, 78.3) -> (17.3, 97) projected
  line L1 (17.3, 97) -> (-15, 97) projected
  line L2 (-15, 97) -> (-15, 78.3) projected
  line L3 (-15, 78.3) -> (17.3, 78.3) projected
  line L4 (12.24, 7) -> (12.24, 22.5) projected
  line L5 (12.24, 22.5) -> (-7, 22.5) projected
  line L6 (-7, 22.5) -> (-7, 7) projected
  line L7 (-7, 7) -> (12.24, 7) projected
  line L8 (150.4, 110.9) -> (150.4, 105.9) projected
  line L9 (150.4, 105.9) -> (130.4, 105.9) projected
  line L10 (130.4, 105.9) -> (130.4, 110.9) projected
  line L11 (130.4, 110.9) -> (150.4, 110.9) projected
  circle A0 centre (124.902, 56.094) radius 1 projected
  circle A1 centre (89.469, 56.094) radius 1 projected
  circle A2 centre (89.469, 91.502) radius 1 projected
  circle A3 centre (124.902, 91.502) radius 1 projected
  circle A4 centre (104.2, 13.0337) radius 1.5 projected
  circle A5 centre (46.2, 13.0337) radius 1.5 projected
  circle A6 centre (46.2, 36.0337) radius 1.5 projected
  circle A7 centre (104.2, 36.0337) radius 1.5 projected
  circle A8 centre (104.2, 13.0337) radius 3 projected
  circle A9 centre (46.2, 13.0337) radius 3 projected
  circle A10 centre (104.2, 36.0337) radius 3 projected
  circle A11 centre (46.2, 36.0337) radius 3 projected
  circle A12 centre (-2.46, 5.26) radius 1.275 projected
  circle A13 centre (7.7, 5.26) radius 1.275 projected
  line L12 (91.971, 89) -> (91.971, 58.596) projected
  line L13 (91.971, 58.596) -> (102, 58.596) projected
  line L14 (102, 58.596) -> (102, 39.596) projected
  line L15 (102, 39.596) -> (110.4, 39.596) projected
  line L16 (110.4, 39.596) -> (110.4, -1.404) projected
  line L17 (110.4, -1.404) -> (122.4, -1.404) projected
  line L18 (122.4, -1.404) -> (122.4, 56.094) projected
  circle A14 centre (124.902, 56.094) radius 2.502 projected
  line L19 (122.4, 56.094) -> (122.4, 89) projected
  line L20 (122.4, 89) -> (91.971, 89) projected
  circle A15 centre (89.469, 56.094) radius 2.502 projected
  circle A16 centre (124.902, 91.502) radius 2.502 projected
  circle A17 centre (89.469, 91.502) radius 2.502 projected
  line L21 (162.4, 32.95) -> (157.4, 32.95) projected
  line L22 (157.4, 32.95) -> (157.4, 72.95) projected
  line L23 (157.4, 72.95) -> (162.4, 72.95) projected
  line L24 (162.4, 72.95) -> (162.4, 32.95) projected
  line L25 (-12, 72.95) -> (-7, 72.95) projected
  line L26 (-7, 72.95) -> (-7, 32.95) projected
  line L27 (-7, 32.95) -> (-12, 32.95) projected
  line L28 (-12, 32.95) -> (-12, 72.95) projected
  line L29 (20, 110.9) -> (20, 105.9) projected
  line L30 (20, 105.9) -> (0, 105.9) projected
  line L31 (0, 105.9) -> (0, 110.9) projected
  line L32 (0, 110.9) -> (20, 110.9) projected
  line L33 (137.4, 37) -> (137.4, 34) projected
  line L34 (137.4, 34) -> (134.2775, 34) projected
  line L35 (134.2775, 34) -> (134.2775, 37) projected
  line L36 (134.2775, 37) -> (137.4, 37) projected
  line L37 (137.4, 37) -> (140.5225, 37) projected
  line L38 (140.5225, 37) -> (140.5225, 34) projected
  line L39 (140.5225, 34) -> (137.4, 34) projected
  arc A18 (-12, 116) -> (-17, 111) centre (-12, 111) ccw projected
  line L40 (-12, 116) -> (36.4, 116) projected
  line L41 (36.4, 116) -> (36.4, 115.5) projected
  line L42 (36.4, 115.5) -> (37, 115.5) projected
  line L43 (37, 115.5) -> (50.2, 115.5) projected
  line L44 (50.2, 115.5) -> (50.8, 115.5) projected
  line L45 (50.8, 115.5) -> (50.8, 116) projected
  line L46 (50.8, 116) -> (60.4, 116) projected
  line L47 (60.4, 116) -> (60.4, 115.5) projected
  line L48 (60.4, 115.5) -> (61, 115.5) projected
  line L49 (61, 115.5) -> (74.2, 115.5) projected
  line L50 (74.2, 115.5) -> (74.8, 115.5) projected
  line L51 (74.8, 115.5) -> (74.8, 116) projected
  line L52 (74.8, 116) -> (162.4, 116) projected
  arc A19 (167.4, 111) -> (162.4, 116) centre (162.4, 111) ccw projected
  line L53 (167.4, 111) -> (167.4, -3) projected
  arc A20 (162.4, -8) -> (167.4, -3) centre (162.4, -3) ccw projected
  line L54 (162.4, -8) -> (-12, -8) projected
  arc A21 (-17, -3) -> (-12, -8) centre (-12, -3) ccw projected
  line L55 (-17, -3) -> (-17, 111) projected
  line L56 (37, 115.5) -> (37, 102.8) projected
  line L57 (37, 102.8) -> (35.5, 102.8) projected
  line L58 (35.5, 102.8) -> (35.5, 112) projected
  line L59 (35.5, 112) -> (34, 112) projected
  line L60 (34, 112) -> (34, 114) projected
  line L61 (34, 114) -> (22, 114) projected
  line L62 (22, 114) -> (22, 112) projected
  line L63 (22, 112) -> (-12, 112) projected
  arc A22 (-12, 112) -> (-13, 111) centre (-12, 111) ccw projected
  line L64 (-13, 111) -> (-13, 101) projected
  line L65 (-13, 98) -> (-13, 101) projected
  line L66 (50.2, 102.8) -> (50.2, 115.5) projected
  line L67 (51.7, 102.8) -> (50.2, 102.8) projected
  line L68 (51.7, 112) -> (51.7, 102.8) projected
  line L69 (59.5, 112) -> (51.7, 112) projected
  line L70 (59.5, 102.8) -> (59.5, 112) projected
  line L71 (61, 102.8) -> (59.5, 102.8) projected
  line L72 (61, 115.5) -> (61, 102.8) projected
  line L73 (74.2, 102.8) -> (74.2, 115.5) projected
  line L74 (75.7, 102.8) -> (74.2, 102.8) projected
  line L75 (75.7, 112) -> (75.7, 102.8) projected
  line L76 (116.4, 112) -> (75.7, 112) projected
  line L77 (116.4, 112) -> (128.4, 112) projected
  line L78 (162.4, 112) -> (128.4, 112) projected
  arc A23 (163.4, 111) -> (162.4, 112) centre (162.4, 111) ccw projected
  line L79 (163.4, 60) -> (163.4, 111) projected
  line L80 (165.4, 60) -> (163.4, 60) projected
  line L81 (165.4, 48) -> (165.4, 60) projected
  line L82 (163.4, 48) -> (165.4, 48) projected
  line L83 (163.4, 60) -> (163.4, 48) projected
  line L84 (22, 112) -> (34, 112) projected
  line L85 (-13, 101) -> (20.3, 101) projected
  line L86 (20.3, 101) -> (20.3, 74.3) projected
  line L87 (20.3, 74.3) -> (-13, 74.3) projected
  line L88 (-13, 74.3) -> (-13, 77.3) projected
  line L89 (116.4, 114) -> (116.4, 112) projected
  line L90 (128.4, 114) -> (116.4, 114) projected
  line L91 (128.4, 112) -> (128.4, 114) projected
  line L92 (163.4, 32.8951) -> (163.4, 48) projected
  line L93 (165.4, 32.8951) -> (163.4, 32.8951) projected
  line L94 (165.4, -2.2797) -> (165.4, 32.8951) projected
  line L95 (163.4, -2.2797) -> (165.4, -2.2797) projected
  line L96 (163.4, -3) -> (163.4, -2.2797) projected
  arc A24 (162.4, -4) -> (163.4, -3) centre (162.4, -3) ccw projected
  line L97 (150.4, -4) -> (162.4, -4) projected
  line L98 (150.4, 0) -> (150.4, -4) projected
  line L99 (130.4, 0) -> (150.4, 0) projected
  line L100 (130.4, -4) -> (130.4, 0) projected
  line L101 (128.4, -4) -> (130.4, -4) projected
  line L102 (128.4, -4) -> (116.4, -4) projected
  line L103 (34, -4) -> (116.4, -4) projected
  line L104 (34, -4) -> (22, -4) projected
  line L105 (20, -4) -> (22, -4) projected
  line L106 (20, 0) -> (20, -4) projected
  line L107 (0, 0) -> (20, 0) projected
  line L108 (0, -4) -> (0, 0) projected
  line L109 (-12, -4) -> (0, -4) projected
  arc A25 (-13, -3) -> (-12, -4) centre (-12, -3) ccw projected
  line L110 (-13, 48) -> (-13, -3) projected
  line L111 (-13, 48) -> (-13, 60) projected
  line L112 (-13, 74.3) -> (-13, 60) projected
  line L113 (128.4, -6) -> (128.4, -4) projected
  line L114 (116.4, -6) -> (128.4, -6) projected
  line L115 (116.4, -4) -> (116.4, -6) projected
  line L116 (34, -6) -> (34, -4) projected
  line L117 (22, -6) -> (34, -6) projected
  line L118 (22, -4) -> (22, -6) projected
  line L119 (-15, 48) -> (-13, 48) projected
  line L120 (-15, 60) -> (-15, 48) projected
  line L121 (-13, 60) -> (-15, 60) projected
  line L122 (165.4, 60) -> (163.4, 60) projected
  line L123 (163.4, 60) -> (163.4, 48) projected
  line L124 (163.4, 48) -> (165.4, 48) projected
  line L125 (165.4, 48) -> (165.4, 60) projected
  line L126 (34, -4) -> (22, -4) projected
  line L127 (22, -4) -> (22, -6) projected
  line L128 (22, -6) -> (34, -6) projected
  line L129 (34, -6) -> (34, -4) projected
  line L130 (128.4, -4) -> (116.4, -4) projected
  line L131 (116.4, -4) -> (116.4, -6) projected
  line L132 (116.4, -6) -> (128.4, -6) projected
  line L133 (128.4, -6) -> (128.4, -4) projected
  line L134 (22, 112) -> (34, 112) projected
  line L135 (34, 112) -> (34, 114) projected
  line L136 (34, 114) -> (22, 114) projected
  line L137 (22, 114) -> (22, 112) projected
  line L138 (128.4, 114) -> (116.4, 114) projected
  line L139 (116.4, 114) -> (116.4, 112) projected
  line L140 (116.4, 112) -> (128.4, 112) projected
  line L141 (128.4, 112) -> (128.4, 114) projected
  line L142 (-15, 48) -> (-13, 48) projected
  line L143 (-13, 48) -> (-13, 60) projected
  line L144 (-13, 60) -> (-15, 60) projected
  line L145 (-15, 60) -> (-15, 48) projected
  line L146 (-5, 7) -> (10.24, 7) projected
  line L147 (10.24, 20.5) -> (-5, 20.5) projected
  arc A26 (-12, 116) -> (-17, 111) centre (-12, 111) ccw projected
  line L148 (162.4, 116) -> (-12, 116) projected
  arc A27 (167.4, 111) -> (162.4, 116) centre (162.4, 111) ccw projected
  line L149 (167.4, -3) -> (167.4, 111) projected
  arc A28 (162.4, -8) -> (167.4, -3) centre (162.4, -3) ccw projected
  line L150 (-12, -8) -> (162.4, -8) projected
  arc A29 (-17, -3) -> (-12, -8) centre (-12, -3) ccw projected
  line L151 (-17, 111) -> (-17, -3) projected
  line L152 (102, 58.596) -> (102, 39.596) projected
  line L153 (102, 39.596) -> (110.4, 39.596) projected
  line L154 (110.4, 39.596) -> (110.4, -1.404) projected
  line L155 (110.4, -1.404) -> (122.4, -1.404) projected
  line L156 (122.4, -1.404) -> (122.4, 89) projected
  line L157 (122.4, 89) -> (91.971, 89) projected
  line L158 (91.971, 89) -> (91.971, 58.596) projected
  line L159 (91.971, 58.596) -> (102, 58.596) projected
  line L160 (35.5, 102.8) -> (51.7, 102.8)
  line L161 (51.7, 102.8) -> (51.7, 100.8)
  line L162 (51.7, 100.8) -> (35.5, 100.8)
  line L163 (35.5, 100.8) -> (35.5, 102.8)
  line L164 (59.5, 102.8) -> (75.7, 102.8)
  line L165 (75.7, 102.8) -> (75.7, 100.8)
  line L166 (75.7, 100.8) -> (59.5, 100.8)
  line L167 (59.5, 100.8) -> (59.5, 102.8)
  line L168 (-5, 20.5) -> (-5, 7) projected
  line L169 (10.24, 7) -> (10.24, 20.5) projected
  point P0 (75.2, 54)
  point P1 (6.9482, 0)
  dimension "d504" = 2
  dimension "d505" = 2
  constraints: 16 end point, 4 parallel, 2 horizontal, 2 perpendicular, 1 horizontal alignment
  measures "d504" distance of L160.end L161.end
  measures "d505" distance of L164.end L165.end
extrude "Extrusion62" add sketch "Sketch75" along normal blind 1.5 contours L160 L67 L161 L162 L163 L57 | L164 L74 L165 L166 L167 L71
sketch "Sketch76" plane through (-90.2, 3.5, -24.3) normal (0, 1, 0) x (1, 0, 0)
  line L0 (-1, 3) -> (-2, 3) projected
  line L1 (-2, 3) -> (-1, 3)
  line L2 (-1, 3) -> (-1, 14.7)
  line L3 (-1, 14.7) -> (-2, 14.7)
  line L4 (-2, 14.7) -> (-2, 3)
  point P0 (90.2, -24.3)
  constraints: 8 end point, 2 parallel, 1 horizontal, 1 perpendicular
extrude "Extrusion63" add sketch "Sketch76" along normal blind 0.5
sketch "Sketch77" plane through (-90.2, 17, 57) normal (1, 0, 0) x (0, 0, -1)
  line L0 (51, -13) -> (0, -13) projected
  line L1 (75.95, -2.2) -> (35.95, -2.2) projected
  line L2 (35.95, -15) -> (35.95, -2.2) projected
  line L3 (75.95, -15) -> (35.95, -15) projected
  line L4 (75.95, -15) -> (75.95, -2.2) projected
  line L5 (3, -15) -> (3, -2.2) projected
  line L6 (4, -13) -> (5.5, -13)
  line L7 (5.5, -13) -> (5.5, -2)
  line L8 (5.5, -2) -> (4, -2)
  line L9 (4, -2) -> (4, -13)
  line L10 (6, -2) -> (6, -13)
  line L11 (7.5, -2) -> (6, -2)
  line L12 (7.5, -13) -> (7.5, -2)
  line L13 (6, -13) -> (7.5, -13)
  line L14 (8, -2) -> (8, -13)
  line L15 (9.5, -2) -> (8, -2)
  line L16 (9.5, -13) -> (9.5, -2)
  line L17 (8, -13) -> (9.5, -13)
  line L18 (10, -2) -> (10, -13)
  line L19 (11.5, -2) -> (10, -2)
  line L20 (11.5, -13) -> (11.5, -2)
  line L21 (10, -13) -> (11.5, -13)
  line L22 (12, -2) -> (12, -13)
  line L23 (13.5, -2) -> (12, -2)
  line L24 (13.5, -13) -> (13.5, -2)
  line L25 (12, -13) -> (13.5, -13)
  line L26 (14, -2) -> (14, -13)
  line L27 (15.5, -2) -> (14, -2)
  line L28 (15.5, -13) -> (15.5, -2)
  line L29 (14, -13) -> (15.5, -13)
  line L30 (16, -2) -> (16, -13)
  line L31 (17.5, -2) -> (16, -2)
  line L32 (17.5, -13) -> (17.5, -2)
  line L33 (16, -13) -> (17.5, -13)
  line L34 (18, -2) -> (18, -13)
  line L35 (19.5, -2) -> (18, -2)
  line L36 (19.5, -13) -> (19.5, -2)
  line L37 (18, -13) -> (19.5, -13)
  line L38 (20, -2) -> (20, -13)
  line L39 (21.5, -2) -> (20, -2)
  line L40 (21.5, -13) -> (21.5, -2)
  line L41 (20, -13) -> (21.5, -13)
  line L42 (22, -2) -> (22, -13)
  line L43 (23.5, -2) -> (22, -2)
  line L44 (23.5, -13) -> (23.5, -2)
  line L45 (22, -13) -> (23.5, -13)
  line L46 (24, -2) -> (24, -13)
  line L47 (25.5, -2) -> (24, -2)
  line L48 (25.5, -13) -> (25.5, -2)
  line L49 (24, -13) -> (25.5, -13)
  line L50 (26, -2) -> (26, -13)
  line L51 (27.5, -2) -> (26, -2)
  line L52 (27.5, -13) -> (27.5, -2)
  line L53 (26, -13) -> (27.5, -13)
  point P0 (57, -17)
  point P1 (26, -13)
  point P2 (27.5, -13)
  point P3 (24, -13)
  point P4 (25.5, -13)
  point P5 (22, -13)
  point P6 (23.5, -13)
  point P7 (20, -13)
  point P8 (21.5, -13)
  point P9 (18, -13)
  point P10 (19.5, -13)
  point P11 (17.5, -13)
  point P12 (15.5, -13)
  point P13 (12, -13)
  point P14 (13.5, -13)
  point P15 (10, -13)
  point P16 (11.5, -13)
  point P17 (8, -13)
  point P18 (9.5, -13)
  point P19 (6, -13)
  point P20 (7.5, -13)
  point P21 (5.5, -13)
  dimension "d515" = 1.5
  dimension "d516" = 11
  dimension "d517" = 1
  dimension "d520" = 2
  constraints: 96 end point, 44 horizontal alignment, 24 parallel, 22 collinear, 1 horizontal, 1 perpendicular, 2 other
  measures "d515" distance of L7.end L8.end
  measures "d516" distance of L8.end L6.start
  measures "d517" distance between parallel lines of L9 L5
  measures "d520" distance of L8.end L10.start
extrude "Extrusion64" cut sketch "Sketch77" against normal through all contours L0 L50 L51 L52 | L0 L46 L47 L48 | L0 L42 L43 L44 | L0 L38 L39 L40 | L0 L34 L35 L36 | L0 L30 L31 L32 | L0 L26 L27 L28 | L0 L22 L23 L24 | L0 L18 L19 L20 | L0 L14 L15 L16 | L0 L10 L11 L12 | L0 L9 L8 L7
chamfer "Chamfer15" distance 0.4 angle 45 2 edges at (-68.775, 2, 48.74) (-78.935, 2, 48.74)
chamfer "Chamfer16" distance 1 angle 45 6 edges at (-31.6, 2, -46.8) (-7.6, 2, -46.8) (0.5, 2, -52.4) (-23.5, 2, -52.4) (-15.7, 2, -52.4) (-39.7, 2, -52.4)